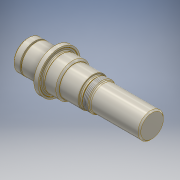
# Autodesk Inventor part: big
Saved by Autodesk Inventor 2016 (Build 200138000, 138)
## iProperties
Created: 2021-04-07
Part Number: big
Material: Типовые
Document SubType Name: Modeling
Designer: Лол
Density: 1 g/cm^3
Appearance: Титан
Author: Лол
Autodesk Inventor part; units mm, degrees
ref_plane "YZ Plane" through (0, 0, 0) normal (1, 0, 0) x (0, 1, 0)
ref_plane "XZ Plane" through (0, 0, 0) normal (0, 1, 0) x (-1, 0, 0)
ref_plane "XY Plane" through (0, 0, 0) normal (0, 0, 1) x (1, 0, 0)
sketch "Эскиз1" plane through (0, 0, 0) normal (0, 0, 1) x (1, 0, 0)
  line L0 (0, 0) -> (0, 17.5)
  line L1 (0, 17.5) -> (8.1, 17.5)
  line L2 (8.1, 17.5) -> (8.1, 15.8)
  line L3 (8.1, 15.8) -> (10, 15.8)
  line L4 (10, 15.8) -> (10, 17.5)
  line L5 (10, 17.5) -> (32, 17.5)
  line L6 (32, 17.5) -> (32, 25)
  line L7 (32, 25) -> (37, 25)
  line L8 (37, 25) -> (37, 20)
  line L9 (79, 17.5) -> (79, 16.5)
  line L10 (79, 16.5) -> (89, 16.5)
  line L11 (89, 16.5) -> (89, 15)
  line L12 (89, 15) -> (147, 15)
  line L13 (147, 15) -> (147, 0)
  line L14 (147, 0) -> (0, 0)
  line L15 (-29.4, 0) -> (176.4, 0) construction
  line L16 (0, -5) -> (0, 30) construction
  line L17 (79, 17.5) -> (55, 17.5)
  line L18 (55, 17.5) -> (55, 20)
  line L19 (55, 20) -> (37, 20)
  point P0 (0, 0)
  point P1 (37, 17.5)
  dimension "d1" = 1.9
  dimension "d2" = 10
  dimension "d3" = 22
  dimension "d4" = 5
  dimension "d6" = 10
  dimension "d7" = 58
  dimension "d12" = 0
  dimension "d13" = 1.7
  dimension "d14" = 0
  dimension "d16" = 35
  dimension "d17" = 50
  dimension "d18" = 33
  dimension "d20" = 30
  dimension "d38" = 17.5
  dimension "d39" = 40
  dimension "d42" = 18
  dimension "d48" = 42
  constraints: 36 end point, 13 perpendicular, 3 point on line, 1 horizontal, 1 vertical
  measures "d1" distance of L2.end L3.end
  measures "d2" distance between parallel lines of L0 L4
  measures "d3" distance of L4.end L5.end
  measures "d4" distance of L6.end L7.end
  measures "d6" distance of L9.end L10.end
  measures "d7" distance of L11.end L12.end
  measures "d12" distance between parallel lines of L0 L16
  measures "d13" distance of L3.end L4.end
  measures "d14" distance between parallel lines of L14 L15
  measures "d16" diameter of L1 L15
  measures "d17" diameter of L7 L15
  measures "d18" diameter of L10 L15
  measures "d20" diameter of L12 L15
  measures "d38" distance between parallel lines of L14 L17
  measures "d39" diameter of L19 L15
  measures "d42" distance of L18.end L8.end
  measures "d48" distance between parallel lines of L8 L9
revolve "Вращение1" add sketch "Эскиз1" angle 360 about axis through (-10, 0, 0) along (1, 0, 0)
thread "Резьба1" size "M33x1.5" class "6g" standard "ANSI Metric M Profile" full length
chamfer "Фаска1" distance 1 angle 45 1 edges at (0, -17.5, 0)
sketch "Эскиз2" plane through (0, 0, 0) normal (0, 0, 1) x (1, 0, 0)
  line L0 (37, -25) -> (37, 25) construction
  line L1 (37, 23.05) -> (36.7, 22.75)
  line L2 (36.7, 22.75) -> (36.7, 19.75)
  line L3 (36.7, 19.75) -> (39.7, 19.75)
  line L4 (39.7, 19.75) -> (39.95, 20)
  line L5 (37, 23.05) -> (39.95, 23.05)
  line L6 (39.95, 23.05) -> (39.95, 20)
  line L7 (-11, 0) -> (66, 0) projected
  line L8 (37, 20) -> (55, 20) construction
  point P0 (0, 0)
  dimension "d28" = 45
  dimension "d29" = 3
  dimension "d31" = 0.3
  dimension "d44" = 45
  dimension "d45" = 0.25
  dimension "d46" = 3.25
  constraints: 12 end point, 4 perpendicular, 1 point on line, 1 vertical
  measures "d28" angle of L0 L1
  measures "d29" distance of L2.end L3.end
  measures "d31" distance between parallel lines of L2 L0
  measures "d44" angle of L8 L4
  measures "d45" distance between parallel lines of L8 L3
  measures "d46" distance between parallel lines of L2 L6
revolve "Вращение2" cut sketch "Эскиз2" angle 360 about axis through (-10, 0, 0) along (1, 0, 0)
fillet "Сопряжение1" radius 1 1 edges at (36.7, -19.75, 0)
fillet "Сопряжение2" radius 0.5 1 edges at (36.7, -22.75, 0)
fillet "Сопряжение3" radius 0.5 1 edges at (39.7, -19.75, 0)
chamfer "Фаска2" distance 2 angle 45 1 edges at (55, -20, 0)
sketch "Эскиз3" plane through (0, 0, 0) normal (0, 0, 1) x (1, 0, 0)
  line L0 (79, -16.5) -> (89, -16.5) construction
  line L1 (79, -17.5) -> (79, 17.5) construction
  line L2 (55, -17.5) -> (79, -17.5) construction
  line L3 (-17.8, 0) -> (106.8, 0) projected
  line L4 (77, -17.5) -> (77, -15.4)
  line L5 (77, -15.4) -> (79.9, -15.4)
  line L6 (79.9, -15.4) -> (81, -16.5)
  line L7 (81, -16.5) -> (81, -20.4)
  line L8 (81, -20.4) -> (77, -20.4)
  line L9 (77, -20.4) -> (77, -17.5)
  point P0 (0, 0)
  dimension "d52" = 45
  dimension "d53" = 4
  dimension "d54" = 15.4
  dimension "d55" = 2
  dimension "d56" = 5
  constraints: 12 end point, 3 perpendicular, 2 point on line, 2 vertical
  measures "d52" angle of L0 L6
  measures "d53" distance between parallel lines of L7 L4
  measures "d54" distance between parallel lines of L3 L5
  measures "d55" distance between parallel lines of L1 L4
  measures "d56" distance between parallel lines of L5 L8
revolve "Вращение3" cut sketch "Эскиз3" angle 360 about axis through (-10, 0, 0) along (1, 0, 0)
fillet "Сопряжение4" radius 1 1 edges at (77, 15.4, 0)
fillet "Сопряжение5" radius 0.5 1 edges at (79.9, 15.4, 0)
chamfer "Фаска3" distance 1.5 angle 45 1 edges at (89, -16.5, 0)
chamfer "Фаска4" distance 1.6 angle 45 1 edges at (147, -15, 0)
fillet "Сопряжение6" radius 2 2 edges at (89, -15, 0) (89, -15.0001, 0)
